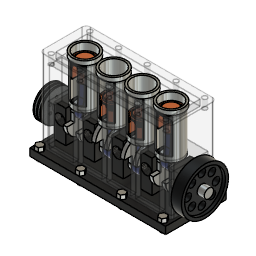
FourCylinderCrankMechanism_2_5D_AI_Model (Autodesk Fusion 360 design; units mm, degrees)
part number: 2026-08-16-04-43-47-560
part number: 2026-08-16-05-09-56-062
part number: 2026-08-16-05-09-56-381
part number: 2026-08-16-05-09-56-439
part number: 2026-08-16-05-09-56-495
part number: 2026-08-16-05-09-56-551
part number: 2026-08-16-05-09-56-611
part number: 2026-08-16-05-09-56-686
part number: 2026-08-16-05-09-57-910
part number: 2026-08-16-05-09-58-143
part number: 2026-08-16-05-09-58-397
part number: 2026-08-16-05-10-47-002
part number: 2026-08-16-05-10-47-440
part number: 2026-08-16-05-10-47-612
part number: 2026-08-16-05-10-47-785
part number: 2026-08-16-05-10-47-965
part number: 2026-08-16-05-10-48-152
part number: 2026-08-16-05-10-48-627
part number: 2026-08-16-05-10-49-092
part number: 2026-08-16-05-10-49-616
part number: 2026-08-16-05-10-50-170
part number: 2026-08-16-05-10-50-272
part number: 2026-08-16-05-10-50-378
part number: 2026-08-16-05-10-50-487
part number: 2026-08-16-05-10-50-594
part number: 2026-08-16-05-10-51-040
part number: 2026-08-16-05-10-51-530
part number: 2026-08-16-05-10-52-032
Autodesk Fusion 360 part; units mm, degrees
sketch "スケッチ1" plane through (0, 0, 0) normal (0, 0, 1) x (1, 0, 0) in component "LowerBedPlate"
  line L0 (-130, -58) -> (130, -58)
  line L1 (130, -58) -> (130, 58)
  line L2 (130, 58) -> (-130, 58)
  line L3 (-130, 58) -> (-130, -58)
extrude "BedPlate_Base" add sketch "スケッチ1" along normal blind 14 from surface at -52 makes body 1 in component "LowerBedPlate"
sketch "スケッチ2" plane through (0, 0, 0) normal (0, 1, 0) x (1, 0, 0) in component "LowerBedPlate"
  line L0 (-121, 42) -> (-99, 42)
  line L1 (-99, 42) -> (-99, -24)
  line L2 (-99, -24) -> (-121, -24)
  line L3 (-121, -24) -> (-121, 42)
  line L4 (-66, 42) -> (-44, 42)
  line L5 (-44, 42) -> (-44, -24)
  line L6 (-44, -24) -> (-66, -24)
  line L7 (-66, -24) -> (-66, 42)
  line L8 (-11, 42) -> (11, 42)
  line L9 (11, 42) -> (11, -24)
  line L10 (11, -24) -> (-11, -24)
  line L11 (-11, -24) -> (-11, 42)
  line L12 (44, 42) -> (66, 42)
  line L13 (66, 42) -> (66, -24)
  line L14 (66, -24) -> (44, -24)
  line L15 (44, -24) -> (44, 42)
  line L16 (99, 42) -> (121, 42)
  line L17 (121, 42) -> (121, -24)
  line L18 (121, -24) -> (99, -24)
  line L19 (99, -24) -> (99, 42)
extrude "BedPlate_Bulkheads (1)" add sketch "スケッチ2" along normal mid plane 40 bodies 1 in component "LowerBedPlate"
sketch "スケッチ3" plane through (0, 0, 0) normal (0, 1, 0) x (1, 0, 0) in component "LowerBedPlate"
  circle A0 centre (-110, 0) radius 10
  circle A1 centre (-55, 0) radius 10
  circle A2 centre (0, 0) radius 10
  circle A3 centre (55, 0) radius 10
  circle A4 centre (110, 0) radius 10
extrude "BedPlate_BearingBores (1)" cut sketch "スケッチ3" along normal mid plane 60 bodies 1 in component "LowerBedPlate"
sketch "スケッチ4" plane through (0, 0, 0) normal (0, 0, 1) x (1, 0, 0) in component "LowerBedPlate"
  circle A0 centre (-118, -51) radius 4.5
extrude "BedPlate_MountHole (1)" cut sketch "スケッチ4" along normal blind 22 from surface at -56 bodies 1 in component "LowerBedPlate"
pattern_linear "BedPlate_MountHolePattern" count 4 spacing 78.6667 along (1, 0, 0) count 3 spacing 0 along (1, 0, 0) of "BedPlate_MountHole (1)" in component "LowerBedPlate"
mirror "BedPlate_MountHoleMirror" about plane through (0, 0, 0) normal (0, 1, 0) of "BedPlate_MountHolePattern" in component "LowerBedPlate"
sketch "スケッチ1 (2)" plane through (0, 0, 0) normal (1, 0, 0) x (0, 0, -1) in component "MainBearing_1"
  circle A0 centre (0, 0) radius 10
  circle A1 centre (0, 0) radius 9.1
extrude "MainBearing_1_Ring" add sketch "スケッチ1 (2)" along normal blind 16 from surface at -118 separate body makes body 2 in component "MainBearing_1"
sketch "スケッチ1 (3)" plane through (0, 0, 0) normal (1, 0, 0) x (0, 0, -1) in component "MainBearing_2"
  circle A0 centre (0, 0) radius 10
  circle A1 centre (0, 0) radius 9.1
extrude "MainBearing_2_Ring" add sketch "スケッチ1 (3)" along normal blind 16 from surface at -63 separate body makes body 3 in component "MainBearing_2"
sketch "スケッチ1 (4)" plane through (0, 0, 0) normal (1, 0, 0) x (0, 0, -1) in component "MainBearing_3"
  circle A0 centre (0, 0) radius 10
  circle A1 centre (0, 0) radius 9.1
extrude "MainBearing_3_Ring" add sketch "スケッチ1 (4)" along normal blind 16 from surface at -8 separate body makes body 4 in component "MainBearing_3"
sketch "スケッチ1 (5)" plane through (0, 0, 0) normal (1, 0, 0) x (0, 0, -1) in component "MainBearing_4"
  circle A0 centre (0, 0) radius 10
  circle A1 centre (0, 0) radius 9.1
extrude "MainBearing_4_Ring" add sketch "スケッチ1 (5)" along normal blind 16 from surface at 47 separate body makes body 5 in component "MainBearing_4"
sketch "スケッチ1 (6)" plane through (0, 0, 0) normal (1, 0, 0) x (0, 0, -1) in component "MainBearing_5"
  circle A0 centre (0, 0) radius 10
  circle A1 centre (0, 0) radius 9.1
extrude "MainBearing_5_Ring" add sketch "スケッチ1 (6)" along normal blind 16 from surface at 102 separate body makes body 6 in component "MainBearing_5"
sketch "スケッチ1 (7)" plane through (0, 0, 0) normal (1, 0, 0) x (0, 0, -1) in component "Crankshaft"
  circle A0 centre (0, 0) radius 9
extrude "Crank_Journal_1 (1)" add sketch "スケッチ1 (7)" along normal blind 23 from surface at -121.5 separate body makes body 7 in component "Crankshaft"
sketch "スケッチ2 (2)" plane through (0, 0, 0) normal (1, 0, 0) x (0, 0, -1) in component "Crankshaft"
  circle A0 centre (0, 0) radius 9
extrude "Crank_Journal_2 (1)" add sketch "スケッチ2 (2)" along normal blind 23 from surface at -66.5 separate body makes body 8 in component "Crankshaft"
sketch "スケッチ3 (2)" plane through (0, 0, 0) normal (1, 0, 0) x (0, 0, -1) in component "Crankshaft"
  circle A0 centre (0, 0) radius 9
extrude "Crank_Journal_3 (1)" add sketch "スケッチ3 (2)" along normal blind 23 from surface at -11.5 separate body makes body 9 in component "Crankshaft"
sketch "スケッチ4 (2)" plane through (0, 0, 0) normal (1, 0, 0) x (0, 0, -1) in component "Crankshaft"
  circle A0 centre (0, 0) radius 9
extrude "Crank_Journal_4 (1)" add sketch "スケッチ4 (2)" along normal blind 23 from surface at 43.5 separate body makes body 10 in component "Crankshaft"
sketch "スケッチ5" plane through (0, 0, 0) normal (1, 0, 0) x (0, 0, -1) in component "Crankshaft"
  circle A0 centre (0, 0) radius 9
extrude "Crank_Journal_5 (1)" add sketch "スケッチ5" along normal blind 23 from surface at 98.5 separate body makes body 11 in component "Crankshaft"
sketch "スケッチ6" plane through (0, 0, 0) normal (1, 0, 0) x (0, 0, -1) in component "Crankshaft"
  circle A0 centre (-18, 0) radius 7
extrude "Crank_Pin_1 (1)" add sketch "スケッチ6" along normal blind 17 from surface at -91 separate body makes body 12 in component "Crankshaft"
sketch "スケッチ7" plane through (0, 0, 0) normal (1, 0, 0) x (0, 0, -1) in component "Crankshaft"
  circle A0 centre (18, 0) radius 7
extrude "Crank_Pin_2 (1)" add sketch "スケッチ7" along normal blind 17 from surface at -36 separate body makes body 13 in component "Crankshaft"
sketch "スケッチ8" plane through (0, 0, 0) normal (1, 0, 0) x (0, 0, -1) in component "Crankshaft"
  circle A0 centre (18, 0) radius 7
extrude "Crank_Pin_3 (1)" add sketch "スケッチ8" along normal blind 17 from surface at 19 separate body makes body 14 in component "Crankshaft"
sketch "スケッチ9" plane through (0, 0, 0) normal (1, 0, 0) x (0, 0, -1) in component "Crankshaft"
  circle A0 centre (-18, 0) radius 7
extrude "Crank_Pin_4 (1)" add sketch "スケッチ9" along normal blind 17 from surface at 74 separate body makes body 15 in component "Crankshaft"
sketch "スケッチ10" plane through (0, 0, 0) normal (1, 0, 0) x (0, 0, -1) in component "Crankshaft"
  arc A0 (0, -26) -> (0, 26) centre (0, 0) ccw
  line L0 (0, 26) -> (0, -26)
  line L1 (6, -11) -> (-18, -11)
  line L2 (-18, -11) -> (-18, 11)
  line L3 (-18, 11) -> (6, 11)
  line L4 (6, 11) -> (6, -11)
  circle A1 centre (-18, 0) radius 11.5
extrude "Crank_Web_1 (1)" add sketch "スケッチ10" along normal blind 7.5 from surface at -98.5 separate body makes body 16 in component "Crankshaft"
sketch "スケッチ11" plane through (0, 0, 0) normal (1, 0, 0) x (0, 0, -1) in component "Crankshaft"
  arc A0 (0, -26) -> (0, 26) centre (0, 0) ccw
  line L0 (0, 26) -> (0, -26)
  line L1 (6, -11) -> (-18, -11)
  line L2 (-18, -11) -> (-18, 11)
  line L3 (-18, 11) -> (6, 11)
  line L4 (6, 11) -> (6, -11)
  circle A1 centre (-18, 0) radius 11.5
extrude "Crank_Web_2 (1)" add sketch "スケッチ11" along normal blind 7.5 from surface at -74 separate body makes body 17 in component "Crankshaft"
sketch "スケッチ12" plane through (0, 0, 0) normal (1, 0, 0) x (0, 0, -1) in component "Crankshaft"
  arc A0 (0, 26) -> (0, -26) centre (0, 0) ccw
  line L0 (0, -26) -> (0, 26)
  line L1 (-6, -11) -> (18, -11)
  line L2 (18, -11) -> (18, 11)
  line L3 (18, 11) -> (-6, 11)
  line L4 (-6, 11) -> (-6, -11)
  circle A1 centre (18, 0) radius 11.5
extrude "Crank_Web_3 (1)" add sketch "スケッチ12" along normal blind 7.5 from surface at -43.5 separate body makes body 18 in component "Crankshaft"
sketch "スケッチ13" plane through (0, 0, 0) normal (1, 0, 0) x (0, 0, -1) in component "Crankshaft"
  arc A0 (0, 26) -> (0, -26) centre (0, 0) ccw
  line L0 (0, -26) -> (0, 26)
  line L1 (-6, -11) -> (18, -11)
  line L2 (18, -11) -> (18, 11)
  line L3 (18, 11) -> (-6, 11)
  line L4 (-6, 11) -> (-6, -11)
  circle A1 centre (18, 0) radius 11.5
extrude "Crank_Web_4 (1)" add sketch "スケッチ13" along normal blind 7.5 from surface at -19 separate body makes body 19 in component "Crankshaft"
sketch "スケッチ14" plane through (0, 0, 0) normal (1, 0, 0) x (0, 0, -1) in component "Crankshaft"
  arc A0 (0, 26) -> (0, -26) centre (0, 0) ccw
  line L0 (0, -26) -> (0, 26)
  line L1 (-6, -11) -> (18, -11)
  line L2 (18, -11) -> (18, 11)
  line L3 (18, 11) -> (-6, 11)
  line L4 (-6, 11) -> (-6, -11)
  circle A1 centre (18, 0) radius 11.5
extrude "Crank_Web_5 (1)" add sketch "スケッチ14" along normal blind 7.5 from surface at 11.5 separate body makes body 20 in component "Crankshaft"
sketch "スケッチ15" plane through (0, 0, 0) normal (1, 0, 0) x (0, 0, -1) in component "Crankshaft"
  arc A0 (0, 26) -> (0, -26) centre (0, 0) ccw
  line L0 (0, -26) -> (0, 26)
  line L1 (-6, -11) -> (18, -11)
  line L2 (18, -11) -> (18, 11)
  line L3 (18, 11) -> (-6, 11)
  line L4 (-6, 11) -> (-6, -11)
  circle A1 centre (18, 0) radius 11.5
extrude "Crank_Web_6 (1)" add sketch "スケッチ15" along normal blind 7.5 from surface at 36 separate body makes body 21 in component "Crankshaft"
sketch "スケッチ16" plane through (0, 0, 0) normal (1, 0, 0) x (0, 0, -1) in component "Crankshaft"
  arc A0 (0, -26) -> (0, 26) centre (0, 0) ccw
  line L0 (0, 26) -> (0, -26)
  line L1 (6, -11) -> (-18, -11)
  line L2 (-18, -11) -> (-18, 11)
  line L3 (-18, 11) -> (6, 11)
  line L4 (6, 11) -> (6, -11)
  circle A1 centre (-18, 0) radius 11.5
extrude "Crank_Web_7 (1)" add sketch "スケッチ16" along normal blind 7.5 from surface at 66.5 separate body makes body 22 in component "Crankshaft"
sketch "スケッチ17" plane through (0, 0, 0) normal (1, 0, 0) x (0, 0, -1) in component "Crankshaft"
  arc A0 (0, -26) -> (0, 26) centre (0, 0) ccw
  line L0 (0, 26) -> (0, -26)
  line L1 (6, -11) -> (-18, -11)
  line L2 (-18, -11) -> (-18, 11)
  line L3 (-18, 11) -> (6, 11)
  line L4 (6, 11) -> (6, -11)
  circle A1 centre (-18, 0) radius 11.5
extrude "Crank_Web_8 (1)" add sketch "スケッチ17" along normal blind 7.5 from surface at 91 separate body makes body 23 in component "Crankshaft"
sketch "スケッチ18" plane through (0, 0, 0) normal (1, 0, 0) x (0, 0, -1) in component "Crankshaft"
  circle A0 centre (0, 0) radius 8
extrude "Crank_FrontNose (1)" add sketch "スケッチ18" along normal blind 33.5 from surface at -155 separate body makes body 24 in component "Crankshaft"
sketch "スケッチ19" plane through (0, 0, 0) normal (1, 0, 0) x (0, 0, -1) in component "Crankshaft"
  circle A0 centre (0, 0) radius 9
extrude "Crank_RearShaft (1)" add sketch "スケッチ19" along normal blind 33.5 from surface at 121.5 separate body makes body 25 in component "Crankshaft"
sketch "スケッチ20" plane through (0, 0, 0) normal (1, 0, 0) x (0, 0, -1) in component "Crankshaft"
  circle A0 centre (0, 0) radius 17
extrude "Crank_RearFlange (1)" add sketch "スケッチ20" along normal blind 8 from surface at 121.5 separate body makes body 26 in component "Crankshaft"
combine "Crankshaft_Combine" operation add target body 7 tool bodies 8 9 10 11 12 13 14 15 16 17 18 19 20 21 22 23 24 25 26 in component "Crankshaft"
sketch "スケッチ1 (8)" plane through (0, 0, 0) normal (0, 1, 0) x (1, 0, 0) in component "Flywheel"
  line L0 (129.5, -9.1) -> (129.5, -39)
  line L1 (129.5, -39) -> (127.5, -39)
  line L2 (127.5, -39) -> (127.5, -45)
  line L3 (127.5, -45) -> (147.5, -45)
  line L4 (147.5, -45) -> (147.5, -39)
  line L5 (147.5, -39) -> (141.5, -39)
  line L6 (141.5, -39) -> (141.5, -9.1)
  line L7 (141.5, -9.1) -> (129.5, -9.1)
revolve "Flywheel_Revolve" add sketch "スケッチ1 (8)" angle 360 about axis through (1.75, 0, 0) along (1, 0, 0) separate body makes body 27 in component "Flywheel"
sketch "スケッチ2 (3)" plane through (0, 0, 0) normal (1, 0, 0) x (0, 0, -1) in component "Flywheel"
  circle A0 centre (-27, 0) radius 7
extrude "Flywheel_LightHole (1)" cut sketch "スケッチ2 (3)" along normal blind 22 from surface at 125 bodies 27 in component "Flywheel"
pattern_circular "Flywheel_LightHolePattern" count 8 over 360 about axis through (1.75, 0, 0) along (1, 0, 0) of "Flywheel_LightHole (1)" in component "Flywheel"
sketch "スケッチ1 (9)" plane through (0, 0, 0) normal (0, 1, 0) x (1, 0, 0) in component "FrontPulley"
  line L0 (-152, -8.1) -> (-152, -30)
  line L1 (-152, -30) -> (-149.5, -30)
  line L2 (-149.5, -30) -> (-148.5, -24)
  line L3 (-148.5, -24) -> (-146.5, -24)
  line L4 (-146.5, -24) -> (-145.5, -30)
  line L5 (-145.5, -30) -> (-143, -30)
  line L6 (-143, -30) -> (-142, -24)
  line L7 (-142, -24) -> (-140, -24)
  line L8 (-140, -24) -> (-139, -30)
  line L9 (-139, -30) -> (-136.5, -30)
  line L10 (-136.5, -30) -> (-136.5, -8.1)
  line L11 (-136.5, -8.1) -> (-152, -8.1)
revolve "FrontPulley_Revolve" add sketch "スケッチ1 (9)" angle 360 about axis through (1.75, 0, 0) along (1, 0, 0) separate body makes body 28 in component "FrontPulley"
sketch "スケッチ2 (4)" plane through (0, 0, 0) normal (1, 0, 0) x (0, 0, -1) in component "FrontPulley"
  circle A0 centre (-14, 0) radius 2.5
extrude "FrontPulley_BoltHole (1)" cut sketch "スケッチ2 (4)" along normal blind 22 from surface at -155 bodies 28 in component "FrontPulley"
pattern_circular "FrontPulley_BoltHolePattern" count 6 over 360 about axis through (1.75, 0, 0) along (1, 0, 0) of "FrontPulley_BoltHole (1)" in component "FrontPulley"
sketch "スケッチ1 (10)" plane through (0, 0, 0) normal (0, 0, 1) x (1, 0, 0) in component "MountBolts"
  circle A0 centre (-118, -51) radius 4.3
extrude "Bolt_Shank (1)" add sketch "スケッチ1 (10)" along normal blind 20 from surface at -56 separate body makes body 29 in component "MountBolts"
sketch "スケッチ2 (5)" plane through (0, 0, 0) normal (0, 0, 1) x (1, 0, 0) in component "MountBolts"
  line L0 (-110.5, -51) -> (-114.25, -44.5048)
  line L1 (-114.25, -44.5048) -> (-121.75, -44.5048)
  line L2 (-121.75, -44.5048) -> (-125.5, -51)
  line L3 (-125.5, -51) -> (-121.75, -57.4952)
  line L4 (-121.75, -57.4952) -> (-114.25, -57.4952)
  line L5 (-114.25, -57.4952) -> (-110.5, -51)
extrude "Bolt_HexHead (1)" add sketch "スケッチ2 (5)" along normal blind 8 from surface at -38 bodies 29 in component "MountBolts"
pattern_linear "MountBolt_Pattern" count 4 spacing 78.6667 along (1, 0, 0) count 2 spacing 102 along (0, 1, 0) of bodies 29 makes body 30 at (-35.0547, -50.5719, -44) makes body 31 at (43.612, -50.5719, -44) makes body 32 at (122.2786, -50.5719, -44) makes body 33 at (-113.7214, 51.4281, -44) makes body 34 at (-35.0547, 51.4281, -44) makes body 35 at (43.612, 51.4281, -44) makes body 36 at (122.2786, 51.4281, -44) in component "MountBolts"
sketch "スケッチ1 (11)" plane through (0, 0, 0) normal (0, 0, 1) x (1, 0, 0) in component "CylinderBlock"
  line L0 (-125, -45) -> (125, -45)
  line L1 (125, -45) -> (125, 45)
  line L2 (125, 45) -> (-125, 45)
  line L3 (-125, 45) -> (-125, -45)
extrude "Block_Base" add sketch "スケッチ1 (11)" along normal blind 156 from surface at -38 separate body makes body 37 in component "CylinderBlock"
sketch "スケッチ2 (6)" plane through (0, 0, 0) normal (0, 0, 1) x (1, 0, 0) in component "CylinderBlock"
  line L0 (-118, -35) -> (118, -35)
  line L1 (118, -35) -> (118, 35)
  line L2 (118, 35) -> (-118, 35)
  line L3 (-118, 35) -> (-118, -35)
extrude "Block_CrankcaseCavity (1)" cut sketch "スケッチ2 (6)" along normal blind 73 from surface at -39 bodies 37 in component "CylinderBlock"
sketch "スケッチ3 (3)" plane through (0, 0, 0) normal (0, 0, 1) x (1, 0, 0) in component "CylinderBlock"
  circle A0 centre (-82.5, 0) radius 22
extrude "Block_Bore (1)" cut sketch "スケッチ3 (3)" along normal blind 90 from surface at 30 bodies 37 in component "CylinderBlock"
pattern_linear "Block_BorePattern" count 4 spacing 55 along (1, 0, 0) count 3 spacing 0 along (1, 0, 0) of "Block_Bore (1)" in component "CylinderBlock"
sketch "スケッチ4 (3)" plane through (0, 0, 0) normal (0, 0, 1) x (1, 0, 0) in component "CylinderBlock"
  line L0 (-105.5, -46) -> (-59.5, -46)
  line L1 (-59.5, -46) -> (-59.5, -21)
  line L2 (-59.5, -21) -> (-105.5, -21)
  line L3 (-105.5, -21) -> (-105.5, -46)
extrude "Block_FrontWindow (1)" cut sketch "スケッチ4 (3)" along normal blind 140 from surface at -34 bodies 37 in component "CylinderBlock"
pattern_linear "Block_FrontWindowPattern" count 4 spacing 55 along (1, 0, 0) count 3 spacing 0 along (1, 0, 0) of "Block_FrontWindow (1)" in component "CylinderBlock"
sketch "スケッチ5 (2)" plane through (0, 0, 0) normal (0, 0, 1) x (1, 0, 0) in component "CylinderBlock"
  line L0 (-108, -30) -> (108, -30)
  line L1 (108, -30) -> (108, 30)
  line L2 (108, 30) -> (-108, 30)
  line L3 (-108, 30) -> (-108, -30)
extrude "Block_TopOpening (1)" cut sketch "スケッチ5 (2)" along normal blind 14 from surface at 106 bodies 37 in component "CylinderBlock"
sketch "スケッチ6 (2)" plane through (0, 0, 0) normal (0, 0, 1) x (1, 0, 0) in component "CylinderBlock"
  circle A0 centre (-110, -37) radius 4.5
extrude "Block_DeckBoltHole (1)" cut sketch "スケッチ6 (2)" along normal blind 20 from surface at 100 bodies 37 in component "CylinderBlock"
pattern_linear "Block_DeckBoltHolePattern" count 5 spacing 55 along (1, 0, 0) count 2 spacing 74 along (0, 1, 0) of "Block_DeckBoltHole (1)" in component "CylinderBlock"
fillet "Block_CornerFillet" radius 8 4 edges at (-125, 45, 40) (125, 45, 40) (125, -45, 40) (-125, -45, 40) on bodies 37 in component "CylinderBlock"
sketch "スケッチ1 (12)" plane through (0, 0, 0) normal (0, 0, 1) x (1, 0, 0) in component "CylinderLiner_1"
  circle A0 centre (-82.5, 0) radius 22
  circle A1 centre (-82.5, 0) radius 20
extrude "Liner_1_Tube" add sketch "スケッチ1 (12)" along normal blind 88 from surface at 30 separate body makes body 38 in component "CylinderLiner_1"
sketch "スケッチ2 (7)" plane through (0, 0, 0) normal (0, 0, 1) x (1, 0, 0) in component "CylinderLiner_1"
  circle A0 centre (-82.5, 0) radius 24
  circle A1 centre (-82.5, 0) radius 20
extrude "Liner_1_Flange (1)" add sketch "スケッチ2 (7)" along normal blind 8 from surface at 110 bodies 38 in component "CylinderLiner_1"
sketch "スケッチ3 (4)" plane through (0, 0, 0) normal (0, 0, 1) x (1, 0, 0) in component "CylinderLiner_1"
  line L0 (-107.5, -30) -> (-57.5, -30)
  line L1 (-57.5, -30) -> (-57.5, -14)
  line L2 (-57.5, -14) -> (-107.5, -14)
  line L3 (-107.5, -14) -> (-107.5, -30)
extrude "Liner_1_ViewWindow (1)" cut sketch "スケッチ3 (4)" along normal blind 68 from surface at 40 bodies 38 in component "CylinderLiner_1"
sketch "スケッチ1 (13)" plane through (0, 0, 0) normal (0, 0, 1) x (1, 0, 0) in component "CylinderLiner_2"
  circle A0 centre (-27.5, 0) radius 22
  circle A1 centre (-27.5, 0) radius 20
extrude "Liner_2_Tube" add sketch "スケッチ1 (13)" along normal blind 88 from surface at 30 separate body makes body 39 in component "CylinderLiner_2"
sketch "スケッチ2 (8)" plane through (0, 0, 0) normal (0, 0, 1) x (1, 0, 0) in component "CylinderLiner_2"
  circle A0 centre (-27.5, 0) radius 24
  circle A1 centre (-27.5, 0) radius 20
extrude "Liner_2_Flange (1)" add sketch "スケッチ2 (8)" along normal blind 8 from surface at 110 bodies 39 in component "CylinderLiner_2"
sketch "スケッチ3 (5)" plane through (0, 0, 0) normal (0, 0, 1) x (1, 0, 0) in component "CylinderLiner_2"
  line L0 (-52.5, -30) -> (-2.5, -30)
  line L1 (-2.5, -30) -> (-2.5, -14)
  line L2 (-2.5, -14) -> (-52.5, -14)
  line L3 (-52.5, -14) -> (-52.5, -30)
extrude "Liner_2_ViewWindow (1)" cut sketch "スケッチ3 (5)" along normal blind 68 from surface at 40 bodies 39 in component "CylinderLiner_2"
sketch "スケッチ1 (14)" plane through (0, 0, 0) normal (0, 0, 1) x (1, 0, 0) in component "CylinderLiner_3"
  circle A0 centre (27.5, 0) radius 22
  circle A1 centre (27.5, 0) radius 20
extrude "Liner_3_Tube" add sketch "スケッチ1 (14)" along normal blind 88 from surface at 30 separate body makes body 40 in component "CylinderLiner_3"
sketch "スケッチ2 (9)" plane through (0, 0, 0) normal (0, 0, 1) x (1, 0, 0) in component "CylinderLiner_3"
  circle A0 centre (27.5, 0) radius 24
  circle A1 centre (27.5, 0) radius 20
extrude "Liner_3_Flange (1)" add sketch "スケッチ2 (9)" along normal blind 8 from surface at 110 bodies 40 in component "CylinderLiner_3"
sketch "スケッチ3 (6)" plane through (0, 0, 0) normal (0, 0, 1) x (1, 0, 0) in component "CylinderLiner_3"
  line L0 (2.5, -30) -> (52.5, -30)
  line L1 (52.5, -30) -> (52.5, -14)
  line L2 (52.5, -14) -> (2.5, -14)
  line L3 (2.5, -14) -> (2.5, -30)
extrude "Liner_3_ViewWindow (1)" cut sketch "スケッチ3 (6)" along normal blind 68 from surface at 40 bodies 40 in component "CylinderLiner_3"
sketch "スケッチ1 (15)" plane through (0, 0, 0) normal (0, 0, 1) x (1, 0, 0) in component "CylinderLiner_4"
  circle A0 centre (82.5, 0) radius 22
  circle A1 centre (82.5, 0) radius 20
extrude "Liner_4_Tube" add sketch "スケッチ1 (15)" along normal blind 88 from surface at 30 separate body makes body 41 in component "CylinderLiner_4"
sketch "スケッチ2 (10)" plane through (0, 0, 0) normal (0, 0, 1) x (1, 0, 0) in component "CylinderLiner_4"
  circle A0 centre (82.5, 0) radius 24
  circle A1 centre (82.5, 0) radius 20
extrude "Liner_4_Flange (1)" add sketch "スケッチ2 (10)" along normal blind 8 from surface at 110 bodies 41 in component "CylinderLiner_4"
sketch "スケッチ3 (7)" plane through (0, 0, 0) normal (0, 0, 1) x (1, 0, 0) in component "CylinderLiner_4"
  line L0 (57.5, -30) -> (107.5, -30)
  line L1 (107.5, -30) -> (107.5, -14)
  line L2 (107.5, -14) -> (57.5, -14)
  line L3 (57.5, -14) -> (57.5, -30)
extrude "Liner_4_ViewWindow (1)" cut sketch "スケッチ3 (7)" along normal blind 68 from surface at 40 bodies 41 in component "CylinderLiner_4"
sketch "スケッチ1 (16)" plane through (0, 0, 0) normal (0, 0, 1) x (1, 0, 0) in component "Piston_1"
  circle A0 centre (-82.5, 0) radius 19.7
extrude "Piston_1_Skirt (1)" add sketch "スケッチ1 (16)" along normal blind 28 from surface at 76 separate body makes body 42 in component "Piston_1"
sketch "スケッチ2 (11)" plane through (0, 0, 0) normal (0, 0, 1) x (1, 0, 0) in component "Piston_1"
  circle A0 centre (-82.5, 0) radius 15
extrude "Piston_1_CrownStep (1)" add sketch "スケッチ2 (11)" along normal blind 2 from surface at 104 bodies 42 in component "Piston_1"
sketch "スケッチ3 (8)" plane through (0, 0, 0) normal (0, 0, 1) x (1, 0, 0) in component "Piston_1"
  circle A0 centre (-82.5, 0) radius 20.2
  circle A1 centre (-82.5, 0) radius 17.7
extrude "Piston_1_RingGroove_1 (1)" cut sketch "スケッチ3 (8)" along normal blind 1.6 from surface at 95.4 bodies 42 in component "Piston_1"
sketch "スケッチ4 (4)" plane through (0, 0, 0) normal (0, 0, 1) x (1, 0, 0) in component "Piston_1"
  circle A0 centre (-82.5, 0) radius 20.2
  circle A1 centre (-82.5, 0) radius 17.7
extrude "Piston_1_RingGroove_2 (1)" cut sketch "スケッチ4 (4)" along normal blind 1.6 from surface at 98.4 bodies 42 in component "Piston_1"
sketch "スケッチ5 (3)" plane through (0, 0, 0) normal (0, 0, 1) x (1, 0, 0) in component "Piston_1"
  circle A0 centre (-82.5, 0) radius 20.2
  circle A1 centre (-82.5, 0) radius 17.7
extrude "Piston_1_RingGroove_3 (1)" cut sketch "スケッチ5 (3)" along normal blind 1.6 from surface at 101.4 bodies 42 in component "Piston_1"
sketch "スケッチ6 (3)" plane through (0, 0, 0) normal (0, 0, 1) x (1, 0, 0) in component "Piston_1"
  line L0 (-89.5, -21) -> (-75.5, -21)
  line L1 (-75.5, -21) -> (-75.5, 21)
  line L2 (-75.5, 21) -> (-89.5, 21)
  line L3 (-89.5, 21) -> (-89.5, -21)
extrude "Piston_1_UnderCrownSlot (1)" cut sketch "スケッチ6 (3)" along normal blind 27.5 from surface at 75 bodies 42 in component "Piston_1"
sketch "スケッチ7 (2)" plane through (0, 0, 0) normal (1, 0, 0) x (0, 0, -1) in component "Piston_1"
  circle A0 centre (-93, 0) radius 5.1
extrude "Piston_1_PinBore (1)" cut sketch "スケッチ7 (2)" along normal blind 50 from surface at -107.5 bodies 42 in component "Piston_1"
chamfer "Piston_1_CrownChamfer" distance 1.5 angle 45 1 edges at (-96.4849, -5.4242, 106) on bodies 42 in component "Piston_1"
sketch "スケッチ1 (17)" plane through (0, 0, 0) normal (0, 0, 1) x (1, 0, 0) in component "Piston_2"
  circle A0 centre (-27.5, 0) radius 19.7
extrude "Piston_2_Skirt (1)" add sketch "スケッチ1 (17)" along normal blind 28 from surface at 40 separate body makes body 43 in component "Piston_2"
sketch "スケッチ2 (12)" plane through (0, 0, 0) normal (0, 0, 1) x (1, 0, 0) in component "Piston_2"
  circle A0 centre (-27.5, 0) radius 15
extrude "Piston_2_CrownStep (1)" add sketch "スケッチ2 (12)" along normal blind 2 from surface at 68 bodies 43 in component "Piston_2"
sketch "スケッチ3 (9)" plane through (0, 0, 0) normal (0, 0, 1) x (1, 0, 0) in component "Piston_2"
  circle A0 centre (-27.5, 0) radius 20.2
  circle A1 centre (-27.5, 0) radius 17.7
extrude "Piston_2_RingGroove_1 (1)" cut sketch "スケッチ3 (9)" along normal blind 1.6 from surface at 59.4 bodies 43 in component "Piston_2"
sketch "スケッチ4 (5)" plane through (0, 0, 0) normal (0, 0, 1) x (1, 0, 0) in component "Piston_2"
  circle A0 centre (-27.5, 0) radius 20.2
  circle A1 centre (-27.5, 0) radius 17.7
extrude "Piston_2_RingGroove_2 (1)" cut sketch "スケッチ4 (5)" along normal blind 1.6 from surface at 62.4 bodies 43 in component "Piston_2"
sketch "スケッチ5 (4)" plane through (0, 0, 0) normal (0, 0, 1) x (1, 0, 0) in component "Piston_2"
  circle A0 centre (-27.5, 0) radius 20.2
  circle A1 centre (-27.5, 0) radius 17.7
extrude "Piston_2_RingGroove_3 (1)" cut sketch "スケッチ5 (4)" along normal blind 1.6 from surface at 65.4 bodies 43 in component "Piston_2"
sketch "スケッチ6 (4)" plane through (0, 0, 0) normal (0, 0, 1) x (1, 0, 0) in component "Piston_2"
  line L0 (-34.5, -21) -> (-20.5, -21)
  line L1 (-20.5, -21) -> (-20.5, 21)
  line L2 (-20.5, 21) -> (-34.5, 21)
  line L3 (-34.5, 21) -> (-34.5, -21)
extrude "Piston_2_UnderCrownSlot (1)" cut sketch "スケッチ6 (4)" along normal blind 27.5 from surface at 39 bodies 43 in component "Piston_2"
sketch "スケッチ7 (3)" plane through (0, 0, 0) normal (1, 0, 0) x (0, 0, -1) in component "Piston_2"
  circle A0 centre (-57, 0) radius 5.1
extrude "Piston_2_PinBore (1)" cut sketch "スケッチ7 (3)" along normal blind 50 from surface at -52.5 bodies 43 in component "Piston_2"
chamfer "Piston_2_CrownChamfer" distance 1.5 angle 45 1 edges at (-41.4849, -5.4242, 70) on bodies 43 in component "Piston_2"
sketch "スケッチ1 (18)" plane through (0, 0, 0) normal (0, 0, 1) x (1, 0, 0) in component "Piston_3"
  circle A0 centre (27.5, 0) radius 19.7
extrude "Piston_3_Skirt (1)" add sketch "スケッチ1 (18)" along normal blind 28 from surface at 40 separate body makes body 44 in component "Piston_3"
sketch "スケッチ2 (13)" plane through (0, 0, 0) normal (0, 0, 1) x (1, 0, 0) in component "Piston_3"
  circle A0 centre (27.5, 0) radius 15
extrude "Piston_3_CrownStep (1)" add sketch "スケッチ2 (13)" along normal blind 2 from surface at 68 bodies 44 in component "Piston_3"
sketch "スケッチ3 (10)" plane through (0, 0, 0) normal (0, 0, 1) x (1, 0, 0) in component "Piston_3"
  circle A0 centre (27.5, 0) radius 20.2
  circle A1 centre (27.5, 0) radius 17.7
extrude "Piston_3_RingGroove_1 (1)" cut sketch "スケッチ3 (10)" along normal blind 1.6 from surface at 59.4 bodies 44 in component "Piston_3"
sketch "スケッチ4 (6)" plane through (0, 0, 0) normal (0, 0, 1) x (1, 0, 0) in component "Piston_3"
  circle A0 centre (27.5, 0) radius 20.2
  circle A1 centre (27.5, 0) radius 17.7
extrude "Piston_3_RingGroove_2 (1)" cut sketch "スケッチ4 (6)" along normal blind 1.6 from surface at 62.4 bodies 44 in component "Piston_3"
sketch "スケッチ5 (5)" plane through (0, 0, 0) normal (0, 0, 1) x (1, 0, 0) in component "Piston_3"
  circle A0 centre (27.5, 0) radius 20.2
  circle A1 centre (27.5, 0) radius 17.7
extrude "Piston_3_RingGroove_3 (1)" cut sketch "スケッチ5 (5)" along normal blind 1.6 from surface at 65.4 bodies 44 in component "Piston_3"
sketch "スケッチ6 (5)" plane through (0, 0, 0) normal (0, 0, 1) x (1, 0, 0) in component "Piston_3"
  line L0 (20.5, -21) -> (34.5, -21)
  line L1 (34.5, -21) -> (34.5, 21)
  line L2 (34.5, 21) -> (20.5, 21)
  line L3 (20.5, 21) -> (20.5, -21)
extrude "Piston_3_UnderCrownSlot (1)" cut sketch "スケッチ6 (5)" along normal blind 27.5 from surface at 39 bodies 44 in component "Piston_3"
sketch "スケッチ7 (4)" plane through (0, 0, 0) normal (1, 0, 0) x (0, 0, -1) in component "Piston_3"
  circle A0 centre (-57, 0) radius 5.1
extrude "Piston_3_PinBore (1)" cut sketch "スケッチ7 (4)" along normal blind 50 from surface at 2.5 bodies 44 in component "Piston_3"
chamfer "Piston_3_CrownChamfer" distance 1.5 angle 45 1 edges at (13.5151, -5.4242, 70) on bodies 44 in component "Piston_3"
sketch "スケッチ1 (19)" plane through (0, 0, 0) normal (0, 0, 1) x (1, 0, 0) in component "Piston_4"
  circle A0 centre (82.5, 0) radius 19.7
extrude "Piston_4_Skirt (1)" add sketch "スケッチ1 (19)" along normal blind 28 from surface at 76 separate body makes body 45 in component "Piston_4"
sketch "スケッチ2 (14)" plane through (0, 0, 0) normal (0, 0, 1) x (1, 0, 0) in component "Piston_4"
  circle A0 centre (82.5, 0) radius 15
extrude "Piston_4_CrownStep (1)" add sketch "スケッチ2 (14)" along normal blind 2 from surface at 104 bodies 45 in component "Piston_4"
sketch "スケッチ3 (11)" plane through (0, 0, 0) normal (0, 0, 1) x (1, 0, 0) in component "Piston_4"
  circle A0 centre (82.5, 0) radius 20.2
  circle A1 centre (82.5, 0) radius 17.7
extrude "Piston_4_RingGroove_1 (1)" cut sketch "スケッチ3 (11)" along normal blind 1.6 from surface at 95.4 bodies 45 in component "Piston_4"
sketch "スケッチ4 (7)" plane through (0, 0, 0) normal (0, 0, 1) x (1, 0, 0) in component "Piston_4"
  circle A0 centre (82.5, 0) radius 20.2
  circle A1 centre (82.5, 0) radius 17.7
extrude "Piston_4_RingGroove_2 (1)" cut sketch "スケッチ4 (7)" along normal blind 1.6 from surface at 98.4 bodies 45 in component "Piston_4"
sketch "スケッチ5 (6)" plane through (0, 0, 0) normal (0, 0, 1) x (1, 0, 0) in component "Piston_4"
  circle A0 centre (82.5, 0) radius 20.2
  circle A1 centre (82.5, 0) radius 17.7
extrude "Piston_4_RingGroove_3 (1)" cut sketch "スケッチ5 (6)" along normal blind 1.6 from surface at 101.4 bodies 45 in component "Piston_4"
sketch "スケッチ6 (6)" plane through (0, 0, 0) normal (0, 0, 1) x (1, 0, 0) in component "Piston_4"
  line L0 (75.5, -21) -> (89.5, -21)
  line L1 (89.5, -21) -> (89.5, 21)
  line L2 (89.5, 21) -> (75.5, 21)
  line L3 (75.5, 21) -> (75.5, -21)
extrude "Piston_4_UnderCrownSlot (1)" cut sketch "スケッチ6 (6)" along normal blind 27.5 from surface at 75 bodies 45 in component "Piston_4"
sketch "スケッチ7 (5)" plane through (0, 0, 0) normal (1, 0, 0) x (0, 0, -1) in component "Piston_4"
  circle A0 centre (-93, 0) radius 5.1
extrude "Piston_4_PinBore (1)" cut sketch "スケッチ7 (5)" along normal blind 50 from surface at 57.5 bodies 45 in component "Piston_4"
chamfer "Piston_4_CrownChamfer" distance 1.5 angle 45 1 edges at (68.5151, -5.4242, 106) on bodies 45 in component "Piston_4"
sketch "スケッチ1 (20)" plane through (0, 0, 0) normal (1, 0, 0) x (0, 0, -1) in component "PistonPin_1"
  circle A0 centre (-93, 0) radius 5
  circle A1 centre (-93, 0) radius 3
extrude "PistonPin_1_Tube" add sketch "スケッチ1 (20)" along normal blind 36 from surface at -100.5 separate body makes body 46 in component "PistonPin_1"
sketch "スケッチ1 (21)" plane through (0, 0, 0) normal (1, 0, 0) x (0, 0, -1) in component "PistonPin_2"
  circle A0 centre (-57, 0) radius 5
  circle A1 centre (-57, 0) radius 3
extrude "PistonPin_2_Tube" add sketch "スケッチ1 (21)" along normal blind 36 from surface at -45.5 separate body makes body 47 in component "PistonPin_2"
sketch "スケッチ1 (22)" plane through (0, 0, 0) normal (1, 0, 0) x (0, 0, -1) in component "PistonPin_3"
  circle A0 centre (-57, 0) radius 5
  circle A1 centre (-57, 0) radius 3
extrude "PistonPin_3_Tube" add sketch "スケッチ1 (22)" along normal blind 36 from surface at 9.5 separate body makes body 48 in component "PistonPin_3"
sketch "スケッチ1 (23)" plane through (0, 0, 0) normal (1, 0, 0) x (0, 0, -1) in component "PistonPin_4"
  circle A0 centre (-93, 0) radius 5
  circle A1 centre (-93, 0) radius 3
extrude "PistonPin_4_Tube" add sketch "スケッチ1 (23)" along normal blind 36 from surface at 64.5 separate body makes body 49 in component "PistonPin_4"
sketch "スケッチ1 (24)" plane through (0, 0, 0) normal (1, 0, 0) x (0, 0, -1) in component "ConnectingRod_1"
  circle A0 centre (-18, 0) radius 13
  circle A1 centre (-93, 0) radius 9
  line L0 (-24, -10.5) -> (-43, -6.5)
  line L1 (-43, -6.5) -> (-68, -6)
  line L2 (-68, -6) -> (-88, -7)
  line L3 (-88, -7) -> (-88, 7)
  line L4 (-88, 7) -> (-68, 6)
  line L5 (-68, 6) -> (-43, 6.5)
  line L6 (-43, 6.5) -> (-24, 10.5)
  line L7 (-24, 10.5) -> (-24, -10.5)
extrude "Rod_1_Web" add sketch "スケッチ1 (24)" along normal blind 10 from surface at -87.5 separate body makes body 50 in component "ConnectingRod_1"
sketch "スケッチ2 (15)" plane through (0, 0, 0) normal (1, 0, 0) x (0, 0, -1) in component "ConnectingRod_1"
  circle A0 centre (-18, 0) radius 13
extrude "Rod_1_BigEndBoss (1)" add sketch "スケッチ2 (15)" along normal blind 15 from surface at -90 bodies 50 in component "ConnectingRod_1"
sketch "スケッチ3 (12)" plane through (0, 0, 0) normal (1, 0, 0) x (0, 0, -1) in component "ConnectingRod_1"
  circle A0 centre (-93, 0) radius 9
extrude "Rod_1_SmallEndBoss (1)" add sketch "スケッチ3 (12)" along normal blind 12 from surface at -88.5 bodies 50 in component "ConnectingRod_1"
sketch "スケッチ4 (8)" plane through (0, 0, 0) normal (1, 0, 0) x (0, 0, -1) in component "ConnectingRod_1"
  circle A0 centre (-18, 0) radius 7.05
  circle A1 centre (-93, 0) radius 5.05
extrude "Rod_1_Bores (1)" cut sketch "スケッチ4 (8)" along normal blind 40 from surface at -102.5 bodies 50 in component "ConnectingRod_1"
sketch "スケッチ1 (25)" plane through (0, 0, 0) normal (1, 0, 0) x (0, 0, -1) in component "ConnectingRod_2"
  circle A0 centre (18, 0) radius 13
  circle A1 centre (-57, 0) radius 9
  line L0 (12, -10.5) -> (-7, -6.5)
  line L1 (-7, -6.5) -> (-32, -6)
  line L2 (-32, -6) -> (-52, -7)
  line L3 (-52, -7) -> (-52, 7)
  line L4 (-52, 7) -> (-32, 6)
  line L5 (-32, 6) -> (-7, 6.5)
  line L6 (-7, 6.5) -> (12, 10.5)
  line L7 (12, 10.5) -> (12, -10.5)
extrude "Rod_2_Web" add sketch "スケッチ1 (25)" along normal blind 10 from surface at -32.5 separate body makes body 51 in component "ConnectingRod_2"
sketch "スケッチ2 (16)" plane through (0, 0, 0) normal (1, 0, 0) x (0, 0, -1) in component "ConnectingRod_2"
  circle A0 centre (18, 0) radius 13
extrude "Rod_2_BigEndBoss (1)" add sketch "スケッチ2 (16)" along normal blind 15 from surface at -35 bodies 51 in component "ConnectingRod_2"
sketch "スケッチ3 (13)" plane through (0, 0, 0) normal (1, 0, 0) x (0, 0, -1) in component "ConnectingRod_2"
  circle A0 centre (-57, 0) radius 9
extrude "Rod_2_SmallEndBoss (1)" add sketch "スケッチ3 (13)" along normal blind 12 from surface at -33.5 bodies 51 in component "ConnectingRod_2"
sketch "スケッチ4 (9)" plane through (0, 0, 0) normal (1, 0, 0) x (0, 0, -1) in component "ConnectingRod_2"
  circle A0 centre (18, 0) radius 7.05
  circle A1 centre (-57, 0) radius 5.05
extrude "Rod_2_Bores (1)" cut sketch "スケッチ4 (9)" along normal blind 40 from surface at -47.5 bodies 51 in component "ConnectingRod_2"
sketch "スケッチ1 (26)" plane through (0, 0, 0) normal (1, 0, 0) x (0, 0, -1) in component "ConnectingRod_3"
  circle A0 centre (18, 0) radius 13
  circle A1 centre (-57, 0) radius 9
  line L0 (12, -10.5) -> (-7, -6.5)
  line L1 (-7, -6.5) -> (-32, -6)
  line L2 (-32, -6) -> (-52, -7)
  line L3 (-52, -7) -> (-52, 7)
  line L4 (-52, 7) -> (-32, 6)
  line L5 (-32, 6) -> (-7, 6.5)
  line L6 (-7, 6.5) -> (12, 10.5)
  line L7 (12, 10.5) -> (12, -10.5)
extrude "Rod_3_Web" add sketch "スケッチ1 (26)" along normal blind 10 from surface at 22.5 separate body makes body 52 in component "ConnectingRod_3"
sketch "スケッチ2 (17)" plane through (0, 0, 0) normal (1, 0, 0) x (0, 0, -1) in component "ConnectingRod_3"
  circle A0 centre (18, 0) radius 13
extrude "Rod_3_BigEndBoss (1)" add sketch "スケッチ2 (17)" along normal blind 15 from surface at 20 bodies 52 in component "ConnectingRod_3"
sketch "スケッチ3 (14)" plane through (0, 0, 0) normal (1, 0, 0) x (0, 0, -1) in component "ConnectingRod_3"
  circle A0 centre (-57, 0) radius 9
extrude "Rod_3_SmallEndBoss (1)" add sketch "スケッチ3 (14)" along normal blind 12 from surface at 21.5 bodies 52 in component "ConnectingRod_3"
sketch "スケッチ4 (10)" plane through (0, 0, 0) normal (1, 0, 0) x (0, 0, -1) in component "ConnectingRod_3"
  circle A0 centre (18, 0) radius 7.05
  circle A1 centre (-57, 0) radius 5.05
extrude "Rod_3_Bores (1)" cut sketch "スケッチ4 (10)" along normal blind 40 from surface at 7.5 bodies 52 in component "ConnectingRod_3"
sketch "スケッチ1 (27)" plane through (0, 0, 0) normal (1, 0, 0) x (0, 0, -1) in component "ConnectingRod_4"
  circle A0 centre (-18, 0) radius 13
  circle A1 centre (-93, 0) radius 9
  line L0 (-24, -10.5) -> (-43, -6.5)
  line L1 (-43, -6.5) -> (-68, -6)
  line L2 (-68, -6) -> (-88, -7)
  line L3 (-88, -7) -> (-88, 7)
  line L4 (-88, 7) -> (-68, 6)
  line L5 (-68, 6) -> (-43, 6.5)
  line L6 (-43, 6.5) -> (-24, 10.5)
  line L7 (-24, 10.5) -> (-24, -10.5)
extrude "Rod_4_Web" add sketch "スケッチ1 (27)" along normal blind 10 from surface at 77.5 separate body makes body 53 in component "ConnectingRod_4"
sketch "スケッチ2 (18)" plane through (0, 0, 0) normal (1, 0, 0) x (0, 0, -1) in component "ConnectingRod_4"
  circle A0 centre (-18, 0) radius 13
extrude "Rod_4_BigEndBoss (1)" add sketch "スケッチ2 (18)" along normal blind 15 from surface at 75 bodies 53 in component "ConnectingRod_4"
sketch "スケッチ3 (15)" plane through (0, 0, 0) normal (1, 0, 0) x (0, 0, -1) in component "ConnectingRod_4"
  circle A0 centre (-93, 0) radius 9
extrude "Rod_4_SmallEndBoss (1)" add sketch "スケッチ3 (15)" along normal blind 12 from surface at 76.5 bodies 53 in component "ConnectingRod_4"
sketch "スケッチ4 (11)" plane through (0, 0, 0) normal (1, 0, 0) x (0, 0, -1) in component "ConnectingRod_4"
  circle A0 centre (-18, 0) radius 7.05
  circle A1 centre (-93, 0) radius 5.05
extrude "Rod_4_Bores (1)" cut sketch "スケッチ4 (11)" along normal blind 40 from surface at 62.5 bodies 53 in component "ConnectingRod_4"
component "LowerBedPlate" placed x (1, 0, 0) y (0, 1, 0) z (0, 0, 1) at (0, 0, 0)
component "MainBearing_1" placed x (1, 0, 0) y (0, 1, 0) z (0, 0, 1) at (0, 0, 0)
component "MainBearing_2" placed x (1, 0, 0) y (0, 1, 0) z (0, 0, 1) at (0, 0, 0)
component "MainBearing_3" placed x (1, 0, 0) y (0, 1, 0) z (0, 0, 1) at (0, 0, 0)
component "MainBearing_4" placed x (1, 0, 0) y (0, 1, 0) z (0, 0, 1) at (0, 0, 0)
component "MainBearing_5" placed x (1, 0, 0) y (0, 1, 0) z (0, 0, 1) at (0, 0, 0)
component "Crankshaft" placed x (1, 0, 0) y (0, 1, 0) z (0, 0, 1) at (0, 0, 0)
component "Flywheel" placed x (1, 0, 0) y (0, 1, 0) z (0, 0, 1) at (0, 0, 0)
component "FrontPulley" placed x (1, 0, 0) y (0, 1, 0) z (0, 0, 1) at (0, 0, 0)
component "MountBolts" placed x (1, 0, 0) y (0, 1, 0) z (0, 0, 1) at (0, 0, 0)
component "CylinderBlock" placed x (1, 0, 0) y (0, 1, 0) z (0, 0, 1) at (0, 0, 0)
component "CylinderLiner_1" placed x (1, 0, 0) y (0, 1, 0) z (0, 0, 1) at (0, 0, 0)
component "CylinderLiner_2" placed x (1, 0, 0) y (0, 1, 0) z (0, 0, 1) at (0, 0, 0)
component "CylinderLiner_3" placed x (1, 0, 0) y (0, 1, 0) z (0, 0, 1) at (0, 0, 0)
component "CylinderLiner_4" placed x (1, 0, 0) y (0, 1, 0) z (0, 0, 1) at (0, 0, 0)
component "Piston_1" placed x (1, 0, 0) y (0, 1, 0) z (0, 0, 1) at (0, 0, 0)
component "Piston_2" placed x (1, 0, 0) y (0, 1, 0) z (0, 0, 1) at (0, 0, 0)
component "Piston_3" placed x (1, 0, 0) y (0, 1, 0) z (0, 0, 1) at (0, 0, 0)
component "Piston_4" placed x (1, 0, 0) y (0, 1, 0) z (0, 0, 1) at (0, 0, 0)
component "PistonPin_1" placed x (1, 0, 0) y (0, 1, 0) z (0, 0, 1) at (0, 0, 0)
component "PistonPin_2" placed x (1, 0, 0) y (0, 1, 0) z (0, 0, 1) at (0, 0, 0)
component "PistonPin_3" placed x (1, 0, 0) y (0, 1, 0) z (0, 0, 1) at (0, 0, 0)
component "PistonPin_4" placed x (1, 0, 0) y (0, 1, 0) z (0, 0, 1) at (0, 0, 0)
component "ConnectingRod_1" placed x (1, 0, 0) y (0, 1, 0) z (0, 0, 1) at (0, 0, 0)
component "ConnectingRod_2" placed x (1, 0, 0) y (0, 1, 0) z (0, 0, 1) at (0, 0, 0)
component "ConnectingRod_3" placed x (1, 0, 0) y (0, 1, 0) z (0, 0, 1) at (0, 0, 0)
component "ConnectingRod_4" placed x (1, 0, 0) y (0, 1, 0) z (0, 0, 1) at (0, 0, 0)
equation "cylinderBore = 40 mm"
equation "cylinderSpacing = 55 mm"
equation "stroke = 36 mm"
equation "crankRadius = 18 mm"
equation "connectingRodLength = 75 mm"
equation "pistonHeight = 28 mm"
equation "pistonPinDiameter = 10 mm"
equation "crankshaftMainDiameter = 18 mm"
equation "crankPinDiameter = 14 mm"
equation "flywheelDiameter = 90 mm"
equation "flywheelThickness = 12 mm"
equation "blockLength = 250 mm"
equation "blockWidth = 90 mm"
equation "blockHeight = 156 mm"
equation "linerOuterDiameter = 44 mm"
equation "mainJournalSpan = 55 mm"
equation "deckHeight = 118 mm"
named bodies: "LowerBedPlateBody", "MainBearingBody", "CrankshaftBody", "FlywheelBody", "FrontPulleyBody", "BoltBody", "BoltBody (1)", "BoltBody (2)", "BoltBody (3)", "BoltBody (4)", "BoltBody (5)", "BoltBody (6)", "BoltBody (7)", "CylinderBlockBody", "CylinderLinerBody", "PistonBody", "PistonPinBody", "ConnectingRodBody"
